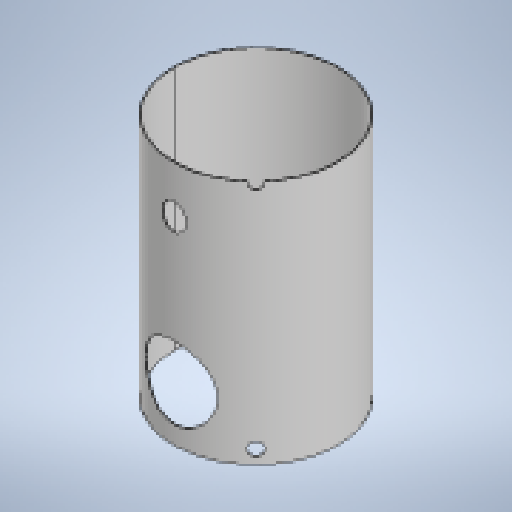
# Autodesk Inventor part: PNS-701 main shell D1200
Saved by Autodesk Inventor 2025.1 (Build 291241020, 241B)
## iProperties
Created: 2025-02-11
Part Number: PNS-701 main shell D1200
Material: Generic
Document SubType Name: Sheet Metal
Designer: pokla
Density: 1 g/cm^3
Flat Pattern Width: 180.342 cm
Flat Pattern Length: 378.545 cm
Flat Pattern Area: 68267.6 cm^2
Sheet Metal Rule: Default_mm
Sheet Metal Width: 1803.422 mm
Sheet Metal Length: 3785.447 mm
Sheet Metal Area: 6826756.915 mm^2
Appearance: Default
Author: pokla
Autodesk Inventor part; units mm, degrees
ref_plane "YZ Plane" through (0, 0, 0) normal (1, 0, 0) x (0, 1, 0)
ref_plane "XZ Plane" through (0, 0, 0) normal (0, 1, 0) x (-1, 0, 0)
ref_plane "XY Plane" through (0, 0, 0) normal (0, 0, 1) x (1, 0, 0)
sketch "Sketch1" plane through (0, 0, 0) normal (0, 1, 0) x (-1, 0, 0)
  line L0 (606, 1803.4216) -> (600, 1803.4216)
  line L1 (600, 1803.4216) -> (600, 0)
  line L2 (600, 0) -> (606, 0)
  line L3 (606, 0) -> (606, 1803.4216)
  line L4 (0, 0) -> (0, 1673.0415)
  point P0 (603, 0)
  dimension "d0" = 6
  dimension "d1" = 1803.4216
  dimension "d2" = 1200
  constraints: 10 end point, 2 parallel, 1 coincident, 1 horizontal, 1 horizontal alignment, 1 midpoint, 1 perpendicular, 1 vertical
  measures "d0" distance between parallel lines of L1 L3
  measures "d1" distance of L2.end L0.start
  measures "d2" diameter of L1 L4
revolve "Revolution1" add sketch "Sketch1" angle 359.9 about axis through (0, 0, 0) along (0, 0, 1)
sketch "Sketch2" plane through (0, 0, 0) normal (0, 1, 0) x (-1, 0, 0)
  circle A0 centre (0, 400) radius 265
  line L0 (600, 1803.4216) -> (-600, 1803.4216) projected
  line L1 (110, 1603.4216) -> (-110, 1603.4216) construction
  line L2 (110, 1693.4216) -> (-110, 1693.4216)
  line L3 (-110, 1513.4216) -> (110, 1513.4216)
  arc A1 (110, 1513.4216) -> (110, 1693.4216) centre (110, 1603.4216) ccw
  arc A2 (-110, 1693.4216) -> (-110, 1513.4216) centre (-110, 1603.4216) ccw
  line L4 (200, 1603.4216) -> (-200, 1603.4216) construction
  point P0 (0, 0)
  point P1 (599.9991, 1803.4216)
  point P2 (0, 1603.4216)
  dimension "d4" = 530
  dimension "d12" = 400
  dimension "d15" = 200
  dimension "d16" = 400
  dimension "d17" = 180
  constraints: 10 end point, 6 point on circle, 4 tangent, 3 centre point, 2 vertical alignment, 1 horizontal, 1 midpoint, 1 parallel
  measures "d4" diameter of A0
  measures "d12" distance of A0.centre point (0, 0)
  measures "d15" distance between parallel lines of L1 L0
  measures "d16" distance of L4.start L4.end
  measures "d17" distance between parallel lines of L3 L2
extrude "Extrusion1" cut sketch "Sketch2" against normal through all contours A0
sketch "Sketch3" plane through (0, 0, 0) normal (0, 0, 1) x (1, 0, 0)
  line L0 (0, 0) -> (0, -267.717)
  line L1 (0, -267.717) -> (0, 0)
  line L2 (0, 0) -> (-190.6162, -190.6162)
  dimension "d18" = 45
  constraints: 6 end point, 1 collinear, 1 vertical
  measures "d18" angle of L0 L2
ref_plane "Work Plane2" through (0, 0, -10) normal (0.7071068, -0.7071068, 0) x (0, 0, 1)
sketch "Sketch4" plane through (0, 0, -10) normal (0.7071068, -0.7071068, 0) x (0, 0, 1)
  circle A0 centre (1810, 0) radius 45
  circle A1 centre (110, 0) radius 47.358
  point P0 (10, 0)
  dimension "d19" = 90
  dimension "d20" = 100
  dimension "d21" = 1800
  constraints: 2 centre point, 2 horizontal alignment
  measures "d19" diameter of A0
  measures "d20" distance of A1.centre point (10, 0)
  measures "d21" distance of A0.centre point (10, 0)
extrude "Extrusion2" cut sketch "Sketch4" along normal through all
sketch "Sketch5" plane through (0, 0, 0) normal (1, 0, 0) x (0, 1, 0)
  line L0 (606, 1803.4216) -> (-606, 1803.4216) projected
  line L1 (-600, 1803.4216) -> (-600, 0) projected
  line L2 (-600, 1453.4216) -> (1.0472, 1106.4069)
  line L3 (1.0472, 0) -> (1.0472, 1803.4216) projected
  point P0 (0, 0)
  point P1 (0, 1803.4216)
  point P2 (1.0577, 1803.4216)
  dimension "d24" = 30
  dimension "d25" = 350
  constraints: 2 end point, 2 point on line
  measures "d24" angle of L2 L0
  measures "d25" distance from line of L2.start L0
ref_plane "Work Plane3" through (0, 1.0472, 1106.4069) normal (0, 0.8660254, -0.5) x (-1, 0, 0)
sketch "Sketch6" plane through (0, 1.0472, 1106.4069) normal (0, 0.8660254, -0.5) x (-1, 0, 0)
  circle A0 centre (0, 0) radius 86
  point P0 (0, -958.7)
  dimension "d26" = 172
  constraints: 1 centre point, 1 coincident
  measures "d26" diameter of A0
extrude "Extrusion3" cut sketch "Sketch6" against normal through all
equation "\"d1\" = MAIN_hight - 2 * Disherd_head_hight"
equation "\"d2\" = MAIN_filter_diam"
equation "\"d4\" = Accsess_hatch_diameter"
equation "\"d16\" = Charging_hatch_width"
equation "\"d17\" = Charging_hatch_hight"
equation "\"BendRadius\" = Thickness"
equation "\"BendReliefWidth\" = Thickness"
equation "\"BendReliefDepth\" = 0.5 * Thickness"
equation "\"CornerReliefSize\" = 4 * Thickness"
equation "\"MinimumRemnant\" = 2 * Thickness"
equation "\"TransitionRadius\" = BendRadius"
equation "\"JacobiRadiusSize\" = BendRadius"
equation "\"GapSize\" = Thickness"
equation "\"MAIN_hight\" = 2310"
equation "\"Disherd_head_hight\" = 253.289193"
equation "\"MAIN_filter_diam\" = 1200"
equation "\"Accsess_hatch_diameter\" = 530"
equation "\"Charging_hatch_width\" = 400"
equation "\"Charging_hatch_hight\" = 180"
equation "\"Thickness\" = 6"
body "Solid1"
